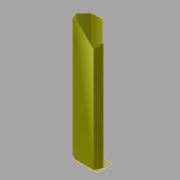
# Autodesk Inventor part: aluco de metro
Saved by Autodesk Inventor 2014 (Build 180170000, 170)
## iProperties
Created: 2016-12-13
Part Number: aluco de metro
Material: Steel, Carbon
Document SubType Name: Modeling
Designer: Cristian
Density: 7.87 g/cm^3
Appearance: Smooth - Yellow
Author: Cristian
Autodesk Inventor part; units mm, degrees
ref_plane "YZ Plane" through (0, 0, 0) normal (1, 0, 0) x (0, 1, 0)
ref_plane "XZ Plane" through (0, 0, 0) normal (0, 1, 0) x (-1, 0, 0)
ref_plane "XY Plane" through (0, 0, 0) normal (0, 0, 1) x (1, 0, 0)
sketch "Sketch1" plane through (0, 0, 0) normal (0, 0, 1) x (1, 0, 0)
  arc A0 (-6.0005, 54.2016) -> (-16.0004, 64.2461) centre (-16.0004, 54.2461) ccw construction
  line L0 (-16.0004, 64.2461) -> (-44.425, 64.2461) construction
  line L1 (-44.425, 64.2461) -> (-109.442, 0.9553) construction
  line L2 (-109.442, 0.9553) -> (-102.1149, -16.5964) construction
  arc A1 (-102.1149, -16.5964) -> (-98.2137, -18.2187) centre (-99.3465, -15.4407) ccw construction
  arc A2 (-98.2137, -18.2187) -> (-94.934, -16.1156) centre (-102.2552, -8.3072) ccw construction
  arc A3 (-90.1342, -27.6135) -> (-94.934, -16.1156) centre (-85.3155, -18.8511) ccw construction
  arc A4 (-90.1342, -27.6135) -> (-93.9357, -28.4666) centre (-89.7305, -38.3096) ccw construction
  arc A5 (-93.9357, -28.4666) -> (-95.5255, -32.381) centre (-92.7571, -31.2253) ccw construction
  line L3 (-95.5255, -32.381) -> (-88, -50.4082) construction
  line L4 (-88, -50.4082) -> (88, -50.4082) construction
  line L5 (88, -50.4082) -> (95.5255, -32.381) construction
  arc A6 (95.5255, -32.381) -> (93.9357, -28.4666) centre (92.7571, -31.2253) ccw construction
  arc A7 (93.9357, -28.4666) -> (90.1342, -27.6135) centre (89.7305, -38.3096) ccw construction
  arc A8 (94.934, -16.1156) -> (90.1342, -27.6135) centre (85.3155, -18.8511) ccw construction
  arc A9 (94.934, -16.1156) -> (98.2137, -18.2187) centre (102.2552, -8.3072) ccw construction
  arc A10 (98.2137, -18.2187) -> (102.1149, -16.5964) centre (99.3465, -15.4407) ccw construction
  line L6 (102.1149, -16.5964) -> (109.442, 0.9553) construction
  line L7 (109.442, 0.9553) -> (44.425, 64.2461) construction
  line L8 (44.425, 64.2461) -> (16.0004, 64.2461) construction
  arc A11 (16.0004, 64.2461) -> (6.0005, 54.2016) centre (16.0004, 54.2461) ccw construction
  arc A12 (6.0005, 54.2016) -> (6.0352, 52.5653) centre (54.7865, 54.419) ccw construction
  arc A13 (-6.0352, 52.5653) -> (6.0352, 52.5653) centre (0, 44.5918) ccw construction
  arc A14 (-6.0352, 52.5653) -> (-6.0005, 54.2016) centre (-54.7865, 54.419) ccw construction
  line L9 (109.442, 0.9553) -> (88, -50.4082)
  line L10 (88, -50.4082) -> (-88, -50.4082)
  line L11 (-88, -50.4082) -> (-109.442, 0.9553)
  line L12 (-109.442, 0.9553) -> (-44.425, 64.2461)
  line L13 (-44.425, 64.2461) -> (-24.425, 64.2461)
  line L14 (109.442, 0.9553) -> (95.1109, 14.9059)
  line L15 (-24.425, 60.2461) -> (-42.7995, 60.2461)
  line L16 (-42.7995, 60.2461) -> (-104.7029, -0.0138)
  line L17 (-104.7029, -0.0138) -> (-85.3353, -46.4082)
  line L18 (-85.3353, -46.4082) -> (85.3353, -46.4082)
  line L19 (85.3353, -46.4082) -> (104.7029, -0.0138)
  line L20 (104.7029, -0.0138) -> (92.3208, 12.0397)
  line L21 (92.3208, 12.0397) -> (95.1109, 14.9059)
  line L22 (-24.425, 60.2461) -> (-24.425, 64.2461)
  point P0 (0, 0)
  dimension "d1" = 20
  dimension "d2" = 20
  dimension "d3" = 4
  constraints: 28 end point, 3 collinear, 2 point on line, 1 horizontal, 1 perpendicular, 1 vertical, 5 other
  measures "d1" distance of L0.end L13.end
  measures "d2" distance of L6.end L14.end
  measures "d3" distance between parallel lines of L4 L18
extrude "Extrusion1" add sketch "Sketch1" along normal blind 1000
ref_plane "Work Plane1" through (0, 0, 0) normal (0, 0, 1) x (1, 0, 0)
sketch "Sketch2" plane through (0, 0, 0) normal (0, 0, 1) x (1, 0, 0)
  line L0 (109.442, 0.9553) -> (44.425, 64.2461) construction
  line L1 (-16.0004, 64.2461) -> (-44.425, 64.2461) projected
  line L2 (-44.425, 64.2461) -> (-109.442, 0.9553) projected
  line L3 (-109.442, 0.9553) -> (-88, -50.4082) projected
  line L4 (-88, -50.4082) -> (88, -50.4082) projected
  line L5 (88, -50.4082) -> (109.442, 0.9553) projected
  line L6 (109.442, 0.9553) -> (95.1109, 14.9059) projected
  line L7 (95.1109, 14.9059) -> (92.3208, 12.0397) projected
  line L8 (92.3208, 12.0397) -> (104.7029, -0.0138) projected
  line L9 (104.7029, -0.0138) -> (85.3353, -46.4082) projected
  line L10 (85.3353, -46.4082) -> (-85.3353, -46.4082) projected
  line L11 (-85.3353, -46.4082) -> (-104.7029, -0.0138) projected
  line L12 (-104.7029, -0.0138) -> (-42.7995, 60.2461) projected
  line L13 (-42.7995, 60.2461) -> (-24.425, 60.2461) projected
  line L14 (-24.425, 60.2461) -> (-24.425, 64.2461) projected
  line L15 (-24.425, 64.2461) -> (-44.425, 64.2461) projected
  line L16 (109.442, 0.9553) -> (44.425, 64.2461)
  line L17 (44.425, 64.2461) -> (-44.425, 64.2461)
  line L18 (-44.425, 68.2461) -> (46.0504, 68.2461)
  line L19 (46.0504, 68.2461) -> (112.2321, 3.8215)
  line L20 (-44.425, 64.2461) -> (-44.425, 68.2461)
  line L21 (112.2321, 3.8215) -> (109.442, 0.9553)
  point P0 (0, 0)
  dimension "d6" = 4
  constraints: 12 end point, 1 collinear, 1 horizontal, 1 perpendicular, 1 vertical, 1 other
  measures "d6" distance between parallel lines of L18 L17
extrude "Extrusion2" add sketch "Sketch2" along normal blind 1000 contours L1 L20 L18 L19 L21 L6 L16 L17
fillet "Fillet1" radius 6 3 edges at (88, -50.4082, 500) (-88, -50.4082, 500) (-109.442, 0.9553, 500)
fillet "Fillet2" radius 6 1 edges at (109.442, 0.9553, 500)
chamfer "Chamfer1" distance 1 angle 45 1 edges at (-44.425, 68.2461, 500)
body "Solid1"
